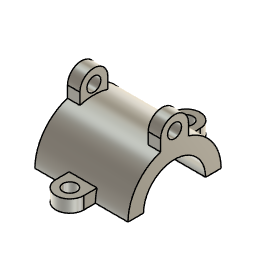
exercise12 (Autodesk Fusion 360 design; units mm, degrees)
Autodesk Fusion 360 part; units mm, degrees
sketch "草图1" plane through (0, 0, 0) normal (1, 0, 0) x (0, 1, 0)
  circle A0 centre (0, 36) radius 4.5
  line L0 (-20, 0) -> (-30, 0)
  line L1 (-30, 0) -> (-46.5, 0)
  line L2 (-46.5, 0) -> (-46.5, 8)
  line L3 (-46.5, 8) -> (-28.9137, 8)
  line L4 (30, 0) -> (46.5, 0)
  line L5 (46.5, 0) -> (46.5, 8)
  line L6 (46.5, 8) -> (28.9137, 8)
  line L7 (30, 0) -> (20, 0)
  arc A1 (30, 0) -> (-30, 0) centre (0, 0) ccw
  arc A2 (20, 0) -> (-20, 0) centre (0, 0) ccw
  line L8 (0, 110) -> (0, -20) construction
  line L9 (-9, 36) -> (-9, 28.6182)
  line L10 (9, 36) -> (9, 28.6182)
  arc A3 (9, 36) -> (-9, 36) centre (0, 36) ccw
  dimension "d1" = 93
  dimension "d2" = 20
  dimension "d3" = 30
  dimension "d4" = 8
  dimension "d5" = 8
  dimension "d6" = 36
  dimension "d7" = 18
  dimension "d8" = 9
  constraint coincident A1.centre A2.centre
  constraint concentric A1 A2
  constraint horizontal L0
  constraint parallel L0 L1
  constraint perpendicular L1 L2
  constraint coincident L3.end A1
  constraint perpendicular L2 L3
  constraint parallel L3 L4
  constraint perpendicular L3 L5
  constraint coincident L6.end A1
  constraint perpendicular L5 L6
  constraint parallel L4 L7
  constraint vertical L8
  constraint coincident A0.centre A3.centre
  constraint coincident A0.centre L8
  constraint coincident A1 L9.end
  constraint vertical L9
  constraint coincident A1 L10.end
  constraint parallel L8 L10
  constraint symmetric L2 L5 L8
  constraint collinear A1.centre L0.end L4.end
  constraint tangent L10 A3
  constraint tangent L9 A3
  measures "d1" distance of L1.end L4.end
  measures "d2" radius of A2
  measures "d3" radius of A1
  measures "d4" distance of L4.end L5.end
  measures "d5" distance of L1.end L2.end
  measures "d6" distance of A1.centre A0.centre
  measures "d7" diameter of A3
  measures "d8" diameter of A0
extrude "拉伸1" add sketch "草图1" along normal mid plane 18 contours L1 L2 L3 A1 | L4 L5 L6 A1 makes body 1 at (-3, 40.6379, 8) makes body 2 at (-3, -40.6379, 8)
extrude "拉伸2" add sketch "草图1" along normal mid plane 60 contours L0 L7 A1 A2 bodies 1 2
extrude "拉伸3" add sketch "草图1" along normal blind 8 separate body contours A1 L9 L10 A3 makes body 3
move_body "移动1" bodies 3 to x (1, 0, 0) y (0, 1, 0) z (0, 0, 1) at (22, 0, 0)
copy_body "复制和粘贴实体1" bodies 3 makes body 4
move_body "移动2" bodies 4 to x (1, 0, 0) y (0, 1, 0) z (0, 0, 1) at (-52, 0, 0)
fillet "圆角1" radius 9 4 edges at (9, -46.5, 4) (-9, -46.5, 4) (9, 46.5, 4) (-9, 46.5, 4) on bodies 1
sketch "草图2" plane through (0, 0, 8) normal (0, 0, 1) x (-1, 0, 0)
  arc A0 (-9, -37.5) -> (9, -37.5) centre (0, -37.5) ccw
  line L0 (9, -37.5) -> (9, -28.9137)
  line L1 (9, -28.9137) -> (-9, -28.9137)
  line L2 (-9, -28.9137) -> (-9, -37.5)
  circle A1 centre (0, -37.5) radius 4.5
  circle A2 centre (0, 37.5) radius 4.5
  line L3 (55, 0) -> (-41.8167, 0) construction
  dimension "d17" = 9
  dimension "d18" = 75
  constraint horizontal L3
  constraint equal A1 A2
  constraint symmetric A0.centre A2.centre L3
  measures "d17" diameter of A1
  measures "d18" distance of A0.centre A2.centre
extrude "拉伸4" cut sketch "草图2" against normal through all contours A1 | A2 bodies 1
combine "合并1" operation add target body 1 tool bodies 4 3
equation "d1 = 75 mm + 18 mm"
